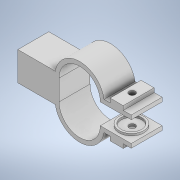
# Autodesk Inventor part: Peça1
Saved by Autodesk Inventor 2022 (Build 260153000, 153)
## iProperties
Created: 2024-03-17
Part Number: Peça1
Material: Genérico
Document SubType Name: Modeling
Designer: Daniel
Density: 1 g/cm^3
Appearance: Padrão
Author: Daniel
Autodesk Inventor part; units mm, degrees
ref_plane "YZ Plane" through (0, 0, 0) normal (1, 0, 0) x (0, 1, 0)
ref_plane "XZ Plane" through (0, 0, 0) normal (0, 1, 0) x (-1, 0, 0)
ref_plane "XY Plane" through (0, 0, 0) normal (0, 0, 1) x (1, 0, 0)
sketch "Esboço1" plane through (0, 0, 0) normal (0, 0, 1) x (1, 0, 0)
  line L0 (0, 0) -> (20, 0)
  arc A0 (40, 0) -> (20, 0) centre (30, 0) ccw
  line L1 (40, 0) -> (55, 0)
  line L2 (55, 2) -> (41.8322, 2)
  arc A1 (41.8322, 2) -> (18.1678, 2) centre (30, 0) ccw
  line L3 (18.1678, 2) -> (0, 2)
  line L4 (0, 0) -> (0, 2)
  line L5 (55, 2) -> (55, 0)
  line L6 (-5.5604, -5) -> (66.7999, -5)
  line L7 (0, -10) -> (20, -10)
  arc A2 (20, -10) -> (40, -10) centre (30, -10) ccw
  line L8 (40, -10) -> (55, -10)
  line L9 (55, -12) -> (41.8322, -12)
  arc A3 (18.1678, -12) -> (41.8322, -12) centre (30, -10) ccw
  line L10 (18.1678, -12) -> (0, -12)
  line L11 (0, -10) -> (0, -12)
  line L12 (55, -12) -> (55, -10)
  line L13 (0, -10) -> (20, -10)
  line L14 (20, -10) -> (20, 0)
  line L15 (20, 0) -> (0, 0)
  line L16 (0, 0) -> (0, -10)
  line L17 (51.1425, 2) -> (44.7734, 2)
  line L18 (44.7734, 2) -> (44.7734, 4)
  line L19 (44.7734, 4) -> (51.1425, 4)
  line L20 (51.1425, 4) -> (51.1425, 2)
  line L21 (51.1425, -12) -> (44.7734, -12)
  line L22 (44.7734, -12) -> (44.7734, -14)
  line L23 (44.7734, -14) -> (51.1425, -14)
  line L24 (51.1425, -14) -> (51.1425, -12)
  dimension "d0" = 20
  dimension "d1" = 20
  dimension "d2" = 10
  dimension "d3" = 15
  dimension "d4" = 2
  dimension "d5" = 10
  dimension "d6" = 2
  dimension "d7" = 2
  constraints: 50 end point, 9 symmetric about line, 8 point on circle, 7 parallel, 6 horizontal, 4 centre point, 4 point on line, 3 perpendicular, 1 vertical, 4 other
  measures "d0" distance of L0.start L0.end
  measures "d1" distance of L0.end L1.start
  measures "d2" radius of A0
  measures "d3" distance of L1.start L1.end
  measures "d4" distance between parallel lines of L1 L2
  measures "d5" diameter of L0 L6
  measures "d6" distance of L19.end L17.start
  measures "d7" distance of L23.end L21.start
extrude "Extrusão1" add sketch "Esboço1" along normal blind 15
sketch "Esboço2" plane through (44.7734, 4, 0) normal (0, 1, 0) x (1, 0, 0)
  circle A0 centre (3.195, -7.5) radius 1.5
  line L0 (6.3691, 0) -> (0, 0) projected
  line L1 (0, 0) -> (0, -15) projected
  point P0 (-44.7734, 0)
  dimension "d10" = 3
  dimension "d11" = 7.5
  dimension "d12" = 3.195
  constraints: 1 centre point
  measures "d10" diameter of A0
  measures "d11" distance from line of L0 A0.centre
  measures "d12" distance from line of L1 A0.centre
extrude "Extrusão2" cut sketch "Esboço2" against normal blind 15
sketch "Esboço3" plane through (40, -10, 0) normal (0, 1, 0) x (1, 0, 0)
  circle A0 centre (7.6045, -7.5) radius 5
  circle A1 centre (7.6045, -7.5) radius 6
  point P0 (-40, 0)
  dimension "d15" = 10
  dimension "d16" = 12
  constraints: 2 centre point, 1 coincident
  measures "d15" diameter of A0
  measures "d16" diameter of A1
extrude "Extrusão3" add sketch "Esboço3" along normal blind 1
sketch "Esboço4" plane through (40, 0, 0) normal (0, -1, 0) x (1, 0, 0)
  circle A0 centre (7.9684, 7.5) radius 1.5 projected
  circle A1 centre (7.9684, 7.5) radius 5
  circle A2 centre (7.9684, 7.5) radius 6
  point P0 (-40, 0)
  dimension "d19" = 10
  dimension "d20" = 12
  constraints: 2 centre point, 2 coincident
  measures "d19" diameter of A1
  measures "d20" diameter of A2
extrude "Extrusão4" add sketch "Esboço4" along normal blind 1 contours A2
